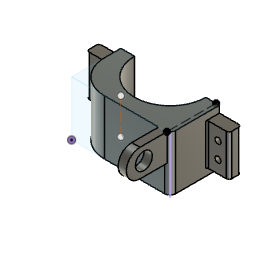
RotaryEncoderModelPole1 (Autodesk Fusion 360 design; units mm, degrees)
Autodesk Fusion 360 part; units mm, degrees
sketch "Sketch1" plane through (0, 0, 0) normal (0, 0, 1) x (1, 0, 0)
  line L0 (0, 0) -> (36, 0)
  line L1 (36, 0) -> (36, 18)
  line L2 (36, 18) -> (0, 18)
  line L3 (0, 18) -> (0, 0)
  dimension "d1" = 36
  dimension "d2" = 18
  constraint coincident L0.start L3.end
  constraint horizontal L0
  constraint perpendicular L0 L1
  constraint perpendicular L1 L2
  constraint perpendicular L0 L3
  measures "d1" distance of L0.start L0.end
  measures "d2" distance of L0.end L1.end
extrude "Extrude1" add sketch "Sketch1" along normal blind 20
sketch "Sketch2" plane through (0, 0, 20) normal (0, 0, 1) x (-1, 0, 0)
  line L0 (0, -18) -> (0, 0)
  line L1 (0, 0) -> (-36, 0)
  line L2 (-36, 0) -> (-36, -18)
  line L3 (-36, -18) -> (0, -18)
  circle A0 centre (-18, -18) radius 13
  dimension "d5" = 26
  constraint midpoint L3 A0.centre
  measures "d5" diameter of A0
extrude "Extrude2" cut sketch "Sketch2" against normal blind 20 contours L3 A0 picked at (-19.0768, -11.2377)
ref_plane "WorkPlane1" through (0, 20, 0) normal (0, 1, 0) x (0, 0, 1)
sketch "Sketch7" plane through (0, 0, 0) normal (0, -1, 0) x (1, 0, 0)
  line L0 (0, 0) -> (36, 0)
  line L1 (36, 20) -> (0, 20)
  line L2 (0, 20) -> (0, 0)
  line L3 (18, 10) -> (18, 23) construction
  line L4 (36, 0) -> (36, 20)
  constraint perpendicular L0 L3
sketch "Sketch6" plane through (36, 0, 0) normal (1, 0, 0) x (0, 1, 0)
  line L0 (0, 0) -> (18, 0)
  line L1 (18, 0) -> (18, 20)
  line L2 (18, 20) -> (0, 20)
  line L3 (0, 20) -> (0, 0)
  line L4 (0, 20) -> (18, 0) construction
  line L5 (0, 0) -> (18, 20) construction
  line L6 (9, 10) -> (18, 10) construction
  line L7 (9, 10) -> (9, 0) construction
  line L8 (9, 10) -> (9, 20) construction
  line L9 (13.5, 17.5) -> (18, 17.5) construction
  line L10 (13.5, 5) -> (13.5, 10) construction
  line L11 (18, 7.5) -> (18, 12.5311)
  line L12 (13.5, 17.5) -> (18, 17.5)
  line L13 (18, 17.5) -> (18, 2.5)
  line L14 (18, 2.5) -> (13.5, 2.5)
  line L15 (13.5, 2.5) -> (13.5, 17.5)
  dimension "d25" = 15
  dimension "d26" = 4.5
  dimension "d34" = 7.5
  constraint coincident L2.end L3.start
  constraint coincident L0.end L1.start
  constraint coincident L0.start L3.end
  constraint coincident L1.end L2.start
  constraint midpoint L5 L6.start
  constraint midpoint L1 L6.end
  constraint perpendicular L6 L7
  constraint midpoint L2 L8.end
  constraint coincident L1 L9.end
  constraint perpendicular L1 L9
  constraint midpoint L6 L10.end
  constraint coincident L1 L11.start
  constraint coincident L1 L11.end
  constraint horizontal L12
  constraint vertical L13
  constraint horizontal L14
  constraint vertical L15
  constraint coincident L1 L13.end
  measures "d25" distance of L9.start L14.end
  measures "d26" distance of L9.start L9.end
  measures "d34" distance of L6 L14
extrude "Extrude7" add sketch "Sketch6" along normal blind 8 contours L1 L11 L12 L13 L14 L15
sketch "Sketch11" plane through (0, 13.5, 0) normal (0, -1, 0) x (1, 0, 0)
  line L0 (36, 17.5) -> (36, 2.5)
  line L1 (36, 2.5) -> (44, 2.5)
  line L2 (44, 2.5) -> (44, 17.5)
  line L3 (44, 17.5) -> (36, 17.5)
  circle A0 centre (40, 13) radius 1.1
  circle A1 centre (40, 7) radius 1.1
  line L4 (36, 0) -> (36, 20)
  line L5 (36, 20) -> (0, 20)
  line L6 (18, 10) -> (18, 23)
  circle A2 centre (-4, 13) radius 1.1
  circle A3 centre (-4, 7) radius 1.1
  dimension "d30" = 2.2
  dimension "d31" = 2.2
  dimension "d35" = 6
  dimension "d36" = 4
  dimension "d37" = 4
  dimension "d38" = 7
  constraint symmetric A0 L6 A2
  constraint symmetric A1 L6 A3
  measures "d30" diameter of A0
  measures "d31" diameter of A1
  measures "d35" vertical distance of A0.centre A1.centre
  measures "d36" distance of A1.centre L4
  measures "d37" distance of A0.centre L4
  measures "d38" distance of A0.centre L5
sketch "Sketch12" plane through (0, 0, 0) normal (-1, 0, 0) x (0, -1, 0)
  line L0 (-18, 0) -> (0, 0)
  line L1 (0, 0) -> (0, 20)
  line L2 (0, 20) -> (-18, 20)
  line L3 (-18, 20) -> (-18, 0)
  line L4 (-18, 17.5) -> (-13.5, 17.5)
  line L5 (-13.5, 17.5) -> (-13.5, 2.5)
  line L6 (-13.5, 2.5) -> (-18, 2.5)
  line L7 (-18, 2.5) -> (-18, 17.5)
  line L8 (-18, 10) -> (-8, 10) construction
  dimension "d39" = 15
  dimension "d40" = 7.5
  dimension "d41" = 4.5
  constraint horizontal L4
  constraint vertical L5
  constraint horizontal L6
  constraint vertical L7
  constraint coincident L3 L4.start
  constraint midpoint L3 L8.start
  constraint perpendicular L7 L8
  measures "d39" distance of L4.end L5.end
  measures "d40" distance of L4 L8
  measures "d41" distance of L4.start L4.end
extrude "Extrude8" add sketch "Sketch12" along normal blind 8 contours L3 L4 L5 L6 L7
extrude "Extrude9" cut sketch "Sketch11" against normal blind 4.5 contours A0 | A1 | A2 | A3
sketch "Sketch13" plane through (0, 0, 20) normal (0, 0, 1) x (-1, 0, 0)
  arc A0 (-5, -18) -> (-31, -18) centre (-18, -18) ccw
  line L0 (-5, -18) -> (0, -18)
  line L1 (0, -18) -> (0, 0)
  line L2 (0, 0) -> (-36, 0)
  line L3 (-36, 0) -> (-36, -18)
  line L4 (-36, -18) -> (-31, -18)
  line L5 (-34.8, -18) -> (-34.8, 0) construction
  dimension "d46" = 3.8
  constraint coincident L4 L5.start
  constraint coincident L2 L5.end
  constraint perpendicular L2 L5
  measures "d46" distance of A0.end L5
sketch "Sketch14" plane through (18, 0, 10) normal (0, -1, 0) x (1, 0, 0)
  line L0 (16.8, 10) -> (13.8, 10)
  line L1 (13.8, 10) -> (13.8, 0)
  line L2 (13.8, 0) -> (16.8, 0)
  line L3 (16.8, 0) -> (16.8, 10)
  point P0 (16.8, 10)
  dimension "d47" = 3
  dimension "d48" = 10
  constraint horizontal L0
  constraint vertical L1
  constraint horizontal L2
  constraint vertical L3
  constraint coincident P0 L0.start
  measures "d47" distance of L1.end L2.end
  measures "d48" distance of L0.end L1.end
extrude "Extrude10" add sketch "Sketch14" along normal blind 14.8
sketch "Sketch15" plane through (34.8, 0, 0) normal (1, 0, 0) x (0, 1, 0)
  line L0 (0, 10) -> (0, 20)
  line L1 (0, 20) -> (-14.8, 20)
  line L2 (-14.8, 20) -> (-14.8, 10)
  line L3 (-14.8, 10) -> (0, 10)
  circle A0 centre (-8.4, 15) radius 3.1
  dimension "d51" = 6.2
  dimension "d52" = 6.4
  dimension "d53" = 5
  measures "d51" diameter of A0
  measures "d52" distance of L2 A0.centre
  measures "d53" distance of L3 A0.centre
extrude "Extrude11" cut sketch "Sketch15" against normal blind 3 contours A0
fillet "Fillet1" radius 5 2 edges at (33.3, -14.8, 20) (33.3, -14.8, 10)
fillet "Fillet2" radius 2 1 edges at (36, 0, 10)
fillet "Fillet3" radius 12 1 edges at (0, 0, 10)
fillet "Fillet4" radius 0.5 1 edges at (0, 13.5, 10)
fillet "Fillet5" radius 1 2 edges at (-8, 18, 10) (-8, 13.5, 10)
fillet "Fillet6" radius 1 2 edges at (44, 13.5, 10) (44, 18, 10)
fillet "Fillet7" radius 0.5 1 edges at (36, 13.5, 10)
fillet "Fillet8" radius 0.5 1 edges at (31.8, 0, 15)
